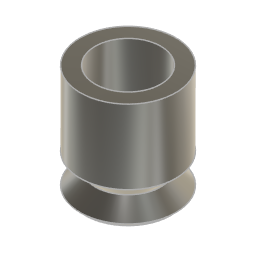
pole-holder_threaded v8 (Autodesk Fusion 360 design; units mm, degrees)
Autodesk Fusion 360 part; units mm, degrees
sketch "Sketch1" plane through (0, 0, 0) normal (0, 0, 1) x (1, 0, 0)
  circle A0 centre (0, 0) radius 6.65
  circle A1 centre (0, 0) radius 9.65
  dimension "d1" = 13.3
  dimension "d2" = 3
  constraint coincident A0.centre A1.centre
  constraint concentric A0 A1
  measures "d1" diameter of A0
  measures "d2" distance of A0 A1
extrude "Extrude1" add sketch "Sketch1" along normal blind 15
extrude "Extrude2" add sketch "Sketch1" along normal blind 5 contours A0
sketch "Sketch2" plane through (0, 0, 0) normal (0, 0, 1) x (1, 0, 0)
  circle A0 centre (0, 0) radius 9.65
  dimension "d7" = 19.3
  constraint coincident A0.centre origin
  measures "d7" diameter of A0
extrude "Extrude3" add sketch "Sketch2" against normal blind 7
sketch "Sketch3" plane through (0, 0, -7) normal (0, 0, -1) x (1, 0, 0)
  circle A0 centre (0, 0) radius 9.65
  circle A1 centre (0, 0) radius 5
  dimension "d10" = 10
  constraint coincident A0.centre A1.centre
  measures "d10" diameter of A1
chamfer "Chamfer1" distance 1 angle 45 1 edges at (-8.997, 3.4896, -7)
sketch "Sketch4" plane through (0, 0, 0) normal (0, 1, 0) x (1, 0, 0)
  line L0 (9.65, 6) -> (-9.65, 6)
  line L1 (9.65, 6) -> (9.65, 0)
  line L2 (9.65, 0) -> (6.65, 3)
  line L3 (6.65, 3) -> (9.65, 6)
  line L4 (0, 0) -> (9.65, 0)
  dimension "d18" = 45
  constraint coincident L0.start L1.start
  constraint equal L2 L3
  constraint coincident L4.start origin
  constraint perpendicular L1 L4
  constraint horizontal L4
  measures "d18" angle of L1 L2
revolve "Revolve1" cut sketch "Sketch4" angle 360 about axis through (0, 0, 1.75) along (0, 0, 1)
